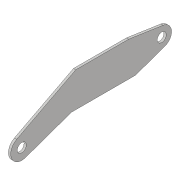
# Autodesk Inventor part: UPPER_LEG_OUTER_FRAME
Saved by Autodesk Inventor 2019.4 (Build 234330000, 330)
## iProperties
Created: 2019-11-12
Part Number: UPPER_LEG_OUTER_FRAME
Material: 一般
Document SubType Name: Modeling
Designer: y6tada
Density: 1 g/cm^3
Appearance: 既定
Author: y6tada
Autodesk Inventor part; units mm, degrees
ref_plane "YZ Plane" through (0, 0, 0) normal (1, 0, 0) x (0, 1, 0)
ref_plane "XZ Plane" through (0, 0, 0) normal (0, 1, 0) x (-1, 0, 0)
ref_plane "XY Plane" through (0, 0, 0) normal (0, 0, 1) x (1, 0, 0)
sketch "スケッチ1" plane through (0, 0, 0) normal (1, 0, 0) x (0, 1, 0)
  circle A0 centre (0, 0) radius 4
  line L0 (0, 0) -> (-22.5, 122.9583) construction
  circle A1 centre (-22.5, 122.9583) radius 4
  line L1 (8.2023, 76.9551) -> (-8.2023, 76.9551) construction
  line L2 (-8.2023, 76.9551) -> (-8.2023, 33.2653) construction
  line L3 (-8.2023, 33.2653) -> (8.2023, 33.2653) construction
  line L4 (8.2023, 33.2653) -> (8.2023, 76.9551) construction
  line L5 (0, 33.2653) -> (0, 0) construction
  line L6 (8.533, -1.2745) -> (13.047, 28.948)
  line L7 (13.047, 28.948) -> (13.047, 75.5059)
  line L8 (13.047, 75.5059) -> (-13.86, 127.4351)
  line L9 (-31.671, 119.7052) -> (-17.3289, 79.2727)
  line L10 (-17.3289, 79.2727) -> (-17.3289, 23.0451)
  line L11 (-17.3289, 23.0451) -> (-8.1312, -2.8843)
  arc A2 (-13.86, 127.4351) -> (-31.671, 119.7052) centre (-22.5, 122.9583) ccw
  arc A3 (-8.1312, -2.8843) -> (8.533, -1.2745) centre (0, 0) ccw
  dimension "d0" = 8
  dimension "d1" = 8
  dimension "d2" = 125
  dimension "d3" = 22.5
  constraints: 24 end point, 4 centre point, 4 point on circle, 4 tangent, 3 parallel, 3 vertical, 2 coincident, 2 concentric, 1 horizontal, 1 midpoint, 1 perpendicular
  measures "d0" diameter of A0
  measures "d1" diameter of A1
  measures "d2" distance of L0.start L0.end
  measures "d3" horizontal distance of point (0, 0) L0.end
extrude "押し出し1" add sketch "スケッチ1" along normal blind 2
